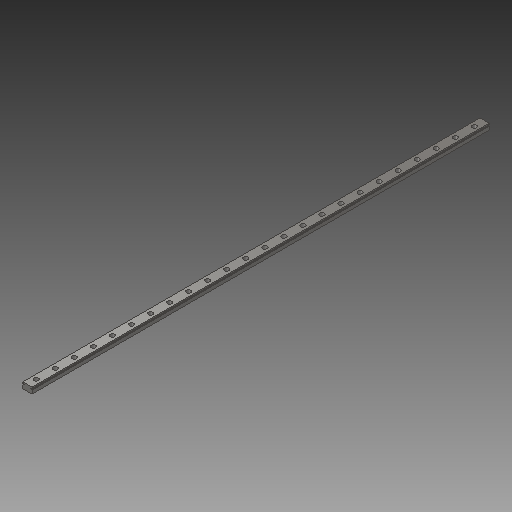
# Autodesk Inventor part: Rail
Saved by Autodesk Inventor 2017 (Build 210142000, 142)
## iProperties
Company: FABLAB Frenchmakers
Part Number: Rail
Material: Acier
Document SubType Name: Modeling
Designer: FABLAB Frenchmakers
Density: 8 g/cm^3
Appearance: Semi-poli(2)
Mass: 405.447 g
Surface Area: 299.353 cm^2
Volume: 50.6809 cm^3
Project: 1420 Vauban 3D XL
Catalog Web Link: http://frenchmakers.com/
Stock Number: 1420-12-01
Autodesk Inventor part; units mm, degrees
ref_plane "YZ Plane" through (0, 0, 0) normal (1, 0, 0) x (0, 1, 0)
ref_plane "XZ Plane" through (0, 0, 0) normal (0, 1, 0) x (-1, 0, 0)
ref_plane "XY Plane" through (0, 0, 0) normal (0, 0, 1) x (1, 0, 0)
sketch "Esquisse1" plane through (0, 0, 0) normal (0, 0, 1) x (1, 0, 0)
  line L0 (-6, -3.95) -> (6, -3.95)
  line L1 (6, -3.95) -> (6, 3.95)
  line L2 (6, 3.95) -> (-6, 3.95)
  line L3 (-6, 3.95) -> (-6, -3.95)
  line L4 (-6, -3.95) -> (6, 3.95) construction
  line L5 (6, -3.95) -> (-6, 3.95) construction
  point P0 (0, 0)
  dimension "d0" = 7.9
  dimension "d1" = 12
  constraints: 12 end point, 2 midpoint, 2 parallel, 1 horizontal, 1 perpendicular
  measures "d0" distance of L2.end L0.start
  measures "d1" distance between parallel lines of L3 L1
extrude "Extrusion1" add sketch "Esquisse1" along normal mid plane 600
sketch "Esquisse2" plane through (0, 0, 300) normal (0, 0, 1) x (1, 0, 0)
  line L0 (6, -3.95) -> (6, 3.95) projected
  line L1 (6, 0.95) -> (4.55, 0.95)
  line L2 (4.3, 1.2) -> (4.3, 1.7)
  line L3 (4.55, 1.95) -> (6, 1.95)
  line L4 (6, 1.95) -> (6, 0.95)
  line L5 (-6, 3.95) -> (-6, -3.95) projected
  line L6 (-6, 0.95) -> (-4.55, 0.95)
  line L7 (-4.3, 1.2) -> (-4.3, 1.7)
  line L8 (-4.55, 1.95) -> (-6, 1.95)
  line L9 (-6, 1.95) -> (-6, 0.95)
  line L10 (-6, 3.95) -> (6, 3.95) projected
  arc A0 (-4.55, 0.95) -> (-4.3, 1.2) centre (-4.55, 1.2) ccw
  arc A1 (-4.3, 1.7) -> (-4.55, 1.95) centre (-4.55, 1.7) ccw
  arc A2 (4.3, 1.2) -> (4.55, 0.95) centre (4.55, 1.2) ccw
  arc A3 (4.55, 1.95) -> (4.3, 1.7) centre (4.55, 1.7) ccw
  point P0 (0, 0)
  point P1 (-4.3, 1.95)
  dimension "d4" = 8.6
  dimension "d5" = 4.3
  dimension "d6" = 1
  dimension "d7" = 2
  dimension "d8" = 0.25
  constraints: 16 end point, 8 point on circle, 8 tangent, 6 point on line, 4 centre point, 4 parallel, 3 equal radius, 2 horizontal, 2 perpendicular
  measures "d4" distance between parallel lines of L2 L7
  measures "d5" distance from line of point (0, 0) L2
  measures "d6" distance between parallel lines of L1 L3
  measures "d7" distance between parallel lines of L10 L3
  measures "d8" radius of A0
extrude "Extrusion2" cut sketch "Esquisse2" against normal through all
fillet "Congé1" radius 0.5 4 edges at (6, 1.95, 0) (6, 0.95, 0) (-6, 0.95, 0) (-6, 1.95, 0)
sketch "Esquisse3" plane through (-6, 3.95, 300) normal (0, 1, 0) x (1, 0, 0)
  line L0 (12, 0) -> (0, 0) projected
  point P0 (6, 300)
  point P1 (6, 11.6)
  dimension "d12" = 11.6
  constraints: 1 vertical alignment
  measures "d12" distance from line of L0 point (6, 11.6)
hole "Perçage1" at (0, 3.95, 288.4) direction (0, -1, 0) diameter 3.5 end through all counterbore diameter 6 counterbore depth 5
pattern_linear "Réseau rectangulaire1" count 24 spacing 25 along (0, 0, -1) of "Perçage1"
equation "\"d5\" = 0.5 * d4"
